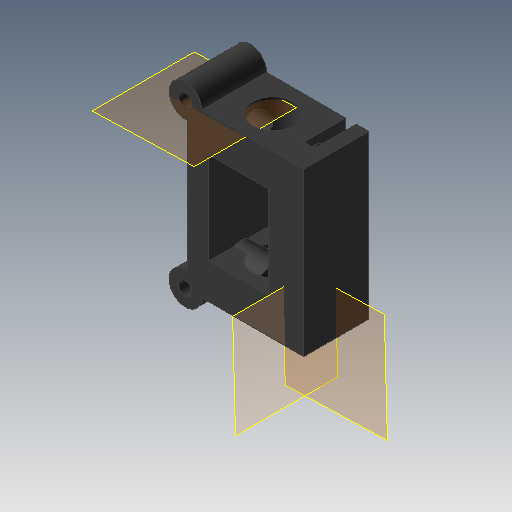
# Autodesk Inventor part: 02_OTmicro_slide_y
Saved by Autodesk Inventor 2019.4 (Build 234330000, 330)
## iProperties
Created: 2020-10-06
Part Number: 02_OTmicro_slide_y
Material: Generic
Document SubType Name: Modeling
Designer: diederichbenedict
Density: 1 g/cm^3
Appearance: Default
Author: diederichbenedict
Autodesk Inventor part; units mm, degrees
ref_plane "YZ Plane" through (0, 0, 0) normal (1, 0, 0) x (0, 1, 0)
ref_plane "XZ Plane" through (0, 0, 0) normal (0, 1, 0) x (-1, 0, 0)
ref_plane "XY Plane" through (0, 0, 0) normal (0, 0, 1) x (1, 0, 0)
ref_plane "Work Plane3" through (0.7186, -2.5999, 12) normal (0, 0, 1) x (0.9996059, 0.0280738, 0)
sketch "Sketch1" plane through (0.7186, -2.5999, 12) normal (0, 0, 1) x (0.9996059, 0.0280738, 0)
  line L0 (-17.6163, 29.2789) -> (-7.6163, 29.2789) projected
  line L1 (-7.6163, 10.3789) -> (-17.6163, 10.3789) projected
  line L2 (-6.7, 17.1444) -> (-6.7, 28.2444)
  line L3 (-18.7, 17.1444) -> (-18.7, 28.2444)
  line L4 (-18.6163, 29.2789) -> (-6.6163, 29.2789) construction
  line L5 (-6.6163, 29.2789) -> (-6.6163, 10.3789) construction
  line L6 (-6.6163, 10.3789) -> (-18.6163, 10.3789) construction
  line L7 (-18.6163, 10.3789) -> (-18.6163, 29.2789) construction
  line L8 (-19.1163, 29.7789) -> (-6.1163, 29.7789)
  line L9 (-6.1163, 29.7789) -> (-6.1163, 9.8789)
  line L10 (-6.1163, 9.8789) -> (-19.1163, 9.8789)
  line L11 (-19.1163, 9.8789) -> (-19.1163, 29.7789)
  line L12 (-19.1163, 29.7789) -> (-6.1163, 9.8789)
  line L13 (-19.1163, 9.8789) -> (-6.1163, 29.7789)
  line L14 (-2.6163, -5.1711) -> (-22.6163, 44.8289) construction
  line L15 (-3.6163, 37.3289) -> (-21.6163, 37.3289)
  line L16 (-21.6163, 37.3289) -> (-21.6163, 2.3289)
  line L17 (-21.6163, 2.3289) -> (-3.6163, 2.3289)
  line L18 (-3.6163, 2.3289) -> (-3.6163, 37.3289)
  line L19 (-3.6163, 37.3289) -> (-21.6163, 2.3289) construction
  line L20 (-21.6163, 37.3289) -> (-3.6163, 2.3289) construction
  line L21 (-21.6163, 2.3289) -> (-23.6163, 2.3289)
  line L22 (-23.6163, 2.3289) -> (-23.6163, 37.3289)
  line L23 (-23.6163, 37.3289) -> (-21.6163, 37.3289)
  line L24 (-21.6163, 37.3289) -> (-21.6163, 2.3289)
  circle A0 centre (-24.1163, 2.3289) radius 2.1 projected
  arc A1 (-24.1163, 39.4289) -> (-24.1163, 35.2289) centre (-24.1163, 37.3289) ccw projected
  arc A2 (-24.1163, 35.2289) -> (-24.1163, 39.4289) centre (-24.1163, 37.3289) ccw projected
  arc A3 (-20.6163, 37.3289) -> (-27.6163, 37.3289) centre (-24.1163, 37.3289) ccw projected
  arc A4 (-27.6163, 2.3289) -> (-20.6163, 2.3289) centre (-24.1163, 2.3289) ccw projected
  circle A5 centre (-24.1163, 2.3289) radius 3.5
  circle A6 centre (-24.1163, 37.3289) radius 3.5
  point P0 (-0.6453, 2.6191)
  point P1 (-12.6163, 19.8289)
  dimension "d0" = 0.5
  dimension "d8" = 18
  dimension "d9" = 35
  dimension "d19" = 9.45
  dimension "d20" = 6
  dimension "d25" = 2
  constraints: 46 end point, 8 parallel, 4 midpoint, 4 perpendicular, 3 horizontal, 2 centre point, 2 coincident, 2 vertical, 1 concentric, 7 other
  measures "d0" distance between parallel lines of L7 L11
  measures "d8" distance of L17.end L16.end
  measures "d9" distance of L16.end L15.end
  measures "d19" distance from line of point (-12.616, 19.829) L1
  measures "d20" distance from line of point (-12.616, 19.829) L7
  measures "d25" distance of L22.end L23.end
extrude "Extrusion1" add sketch "Sketch1" along normal mid plane 14
ref_plane "Work Plane6" through (-22.5262, 34.0909, 19) normal (-0.0280738, 0.9996059, 0) x (0.9996059, 0.0280738, 0)
sketch "Sketch2" plane through (-22.5262, 34.0909, 19) normal (-0.0280738, 0.9996059, 0) x (0.9996059, 0.0280738, 0)
  circle A0 centre (10, 7) radius 4.5
  circle A1 centre (9.5892, 7) radius 3.15 projected
  point P0 (21.5602, 19)
  dimension "d5" = 9
  constraints: 1 centre point
  measures "d5" diameter of A0
extrude "Extrusion2" cut sketch "Sketch2" against normal through all contours A0 | A1
ref_plane "Work Plane7" through (-2.9617, -0.3735, 19) normal (0.9996059, 0.0280738, 0) x (0, 0, -1)
sketch "Sketch3" plane through (-2.9617, -0.3735, 19) normal (0.9996059, 0.0280738, 0) x (0, 0, -1)
  line L0 (0, 35) -> (14, 35) projected
  line L1 (0, 0) -> (0, 35) projected
  line L2 (14, 0) -> (0, 0) projected
  line L3 (14, 35) -> (14, 0) projected
  line L4 (14, 0) -> (0, 0) projected
  line L5 (0, 35) -> (0, 0)
  circle A0 centre (7, 4.8) radius 3.15
  circle A1 centre (7, 30.2) radius 3.15
  line L6 (7, -12.6081) -> (7, 47.131) projected
  point P0 (19, 0.2902)
  dimension "d11" = 6.3
  dimension "d12" = 6.3
  dimension "d22" = 0
  dimension "d23" = 4.8
  dimension "d24" = 4.8
  constraints: 2 centre point, 2 end point
  measures "d11" diameter of A0
  measures "d12" diameter of A1
  measures "d22" distance from line of A0.centre L6
  measures "d23" distance from line of L2 A0.centre
  measures "d24" distance from line of L0 A1.centre
extrude "Extrusion3" cut sketch "Sketch3" against normal through all contours L6 A1 | A1 L6 | L6 A0 | A0 L6
sketch "Sketch4" plane through (0.7186, -2.5999, 19) normal (0, 0, 1) x (0.9996059, 0.0280738, 0)
  arc A0 (-23.6163, 5.793) -> (-20.6163, 2.3289) centre (-24.1163, 2.3289) ccw projected
  arc A1 (-20.6163, 37.3289) -> (-27.6163, 37.3289) centre (-24.1163, 37.3289) ccw projected
  arc A2 (-23.6163, 5.793) -> (-20.6163, 2.3289) centre (-24.1163, 2.3289) ccw projected
  circle A3 centre (-24.1163, 2.3289) radius 1.45
  circle A4 centre (-24.1163, 37.3289) radius 1.45
  point P0 (-0.6453, 2.6191)
  dimension "d26" = 2.9
  dimension "d27" = 2.9
  constraints: 2 centre point, 2 coincident
  measures "d26" diameter of A3
  measures "d27" diameter of A4
extrude "Extrusion4" cut sketch "Sketch4" against normal through all
sketch "Sketch5" plane through (-19.955, -0.8507, 5) normal (0.0280738, -0.9996059, 0) x (0.9996059, 0.0280738, 0)
  line L0 (0, 0) -> (0, 14) projected
  line L1 (17, 0) -> (0, 0) projected
  line L2 (17, 0) -> (17, 14) projected
  line L3 (0, 14) -> (17, 14) projected
  line L4 (17, 0) -> (22, 0)
  line L5 (22, 0) -> (22, 14)
  line L6 (22, 14) -> (17, 14)
  line L7 (17, 14) -> (17, 0)
  line L8 (17, 0) -> (19.3, 0)
  line L9 (19.3, 0) -> (19.3, 9)
  line L10 (19.3, 9) -> (17, 9)
  line L11 (17, 9) -> (17, 0)
  point P0 (19.971, -5)
  dimension "d30" = 5
  dimension "d31" = 2.3
  dimension "d32" = 9
  constraints: 16 end point, 4 parallel, 2 horizontal, 2 perpendicular
  measures "d30" distance of L6.end L5.end
  measures "d31" distance of L10.end L9.end
  measures "d32" distance of L9.end L8.end
extrude "Extrusion5" add sketch "Sketch5" against normal up to surface (35 mm away) contours L6 L5 L4 L9 L10 L2
move or copy body "Move Body1" bodies to move or copy 1 copy no rotation origin (0, 0, 0) rotation axis (0, 0, 1) rotation angle -1.64 translate (-0.9942, 0.0444, 0)
body "Solid1"
